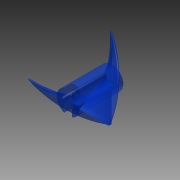
# Autodesk Inventor part: Main Prop
Saved by Autodesk Inventor 2013 (Build 170138000, 138)
## iProperties
Created: 2014-08-02
Part Number: Main Prop
Material: ABS Plastic
Document SubType Name: Modeling
Designer: Kyle
Density: 1 g/cm^3
Author: Kyle
Autodesk Inventor part; units mm, degrees
ref_plane "YZ Plane" through (0, 0, 0) normal (1, 0, 0) x (0, 1, 0)
ref_plane "XZ Plane" through (0, 0, 0) normal (0, 1, 0) x (-1, 0, 0)
sketch "Sketch1" plane through (0, 0, 0) normal (0, 0, 1) x (1, 0, 0)
  circle A0 centre (0, 0) radius 4.0005
  circle A1 centre (0, 0) radius 2.032
  dimension "d0" = 8.001
  dimension "d2" = 4.064
  constraints: 2 centre point, 2 coincident
  measures "d0" diameter of A0
  measures "d2" diameter of A1
extrude "Extrusion1" add sketch "Sketch1" along normal blind 15.24
sketch "Sketch2" plane through (0, 0, 15.24) normal (0, 0, 1) x (1, 0, 0)
  circle A0 centre (0, 0) radius 2.032 projected
  line L0 (-1.397, 5.1605) -> (1.397, 5.1605)
  line L1 (1.397, 5.1605) -> (1.397, -5.4473)
  line L2 (1.397, -5.4473) -> (-1.397, -5.4473)
  line L3 (-1.397, -5.4473) -> (-1.397, 5.1605)
  point P0 (2.032, 5.1605)
  dimension "d5" = 1.397
  dimension "d6" = 1.397
  constraints: 8 end point, 2 parallel, 1 horizontal, 1 perpendicular
  measures "d5" horizontal distance of L0.start A0.centre
  measures "d6" horizontal distance of L1.end A0.centre
extrude "Extrusion2" cut sketch "Sketch2" against normal blind 2.54 contours L1 A0 L3 | A0 L3 L0 L1 | L1 L2 L3 A0
ref_plane "Work Plane1" through (0, 0, 0) normal (0, -1, 0) x (0, 0, -1)
sketch "Sketch3" plane through (0, 0, 0) normal (0, -1, 0) x (0, 0, -1)
  line L0 (-15.24, 4.0005) -> (-15.24, 1.397) projected
  line L1 (-15.24, 4.0005) -> (-14.605, 4.0005)
  line L2 (-14.605, 4.0005) -> (-14.605, 13.9065)
  line L3 (-14.859, 14.1605) -> (-14.986, 14.1605)
  line L4 (-15.24, 13.9065) -> (-15.24, 4.0005)
  arc A0 (-14.986, 14.1605) -> (-15.24, 13.9065) centre (-14.986, 13.9065) ccw
  arc A1 (-14.605, 13.9065) -> (-14.859, 14.1605) centre (-14.859, 13.9065) ccw
  line L5 (-15.24, -4.0005) -> (-14.6794, -4.0005)
  line L6 (-14.6794, -4.0005) -> (-14.6794, -13.9065)
  line L7 (-14.9334, -14.1605) -> (-14.986, -14.1605)
  line L8 (-15.24, -13.9065) -> (-15.24, -4.0005)
  arc A2 (-15.24, -13.9065) -> (-14.986, -14.1605) centre (-14.986, -13.9065) ccw
  arc A3 (-14.9334, -14.1605) -> (-14.6794, -13.9065) centre (-14.9334, -13.9065) ccw
  point P0 (0, 0)
  point P1 (1.7022, 0)
  dimension "d10" = 4.0005
  dimension "d12" = 0.635
  dimension "d13" = 10.16
  dimension "d14" = 0.254
  dimension "d15" = 8.001
  dimension "d16" = 8.001
  dimension "d17" = 10.16
  dimension "d18" = 0.254
  constraints: 16 end point, 8 point on circle, 8 tangent, 4 centre point, 4 parallel, 2 equal radius, 2 horizontal, 2 perpendicular, 1 coincident, 1 other
  measures "d10" vertical distance of point (-14.605, 4.001) point (1.702, 0)
  measures "d12" distance from line of L0 point (-14.605, 4.001)
  measures "d13" distance between parallel lines of L3 L1
  measures "d14" radius of A0
  measures "d15" distance of L1.start L5.start
  measures "d16" vertical distance of L1.start point (-14.679, -4.001)
  measures "d17" distance between parallel lines of L5 L7
  measures "d18" radius of A2
ref_plane "Work Plane2" through (0, 0, 0) normal (-1, 0, 0) x (0, 0, -1)
sketch "Sketch4" plane through (0, 0, 0) normal (-1, 0, 0) x (0, 0, -1)
  line L0 (0, -4.0005) -> (0, 4.0005) projected
  line L1 (-1.9812, -4.0005) -> (-0.0316, -19.5002)
  line L2 (-2.54, -4.0005) -> (-0.5277, -19.5635)
  line L3 (-1.9812, -4.0005) -> (-2.54, -4.0005)
  line L4 (-0.2432, -19.7828) -> (-0.251, -19.7838)
  arc A0 (-0.5277, -19.5635) -> (-0.2432, -19.7828) centre (-0.2757, -19.5309) ccw
  arc A1 (-0.251, -19.7838) -> (-0.0316, -19.5002) centre (-0.2836, -19.5319) ccw
  line L5 (-1.9812, 4.0005) -> (-0.0317, 19.4994)
  line L6 (-2.54, 4.0005) -> (-0.5818, 19.5686)
  line L7 (-0.2981, 19.7889) -> (-0.252, 19.7831)
  arc A2 (-0.0317, 19.4994) -> (-0.252, 19.7831) centre (-0.2837, 19.5311) ccw
  arc A3 (-0.2981, 19.7889) -> (-0.5818, 19.5686) centre (-0.3298, 19.5369) ccw
  line L8 (-2.54, 4.0005) -> (-1.9812, 4.0005)
  point P0 (0, 0)
  point P1 (0.7046, 0)
  point P2 (0, -19.7514)
  point P3 (0, 19.7514)
  dimension "d25" = 15.875
  dimension "d26" = 0
  dimension "d27" = 1.9812
  dimension "d28" = 0.254
  dimension "d29" = 15.875
  dimension "d30" = 0
  dimension "d31" = 1.9812
  dimension "d32" = 0.254
  constraints: 16 end point, 8 point on circle, 8 tangent, 4 centre point, 4 point on line, 3 perpendicular, 2 equal radius, 1 parallel, 1 other
  measures "d25" distance of L1.start point (0, -19.751)
  measures "d26" horizontal distance of L0.start point (0, -19.751)
  measures "d27" distance of L1.start L0.start
  measures "d28" radius of A0
  measures "d29" distance of L5.start point (0, 19.751)
  measures "d30" distance from line of point (0, 19.751) L0
  measures "d31" distance from line of L5.start L0
  measures "d32" radius of A2
coil "Coil1" sketch "Sketch3" operation add axis through (0, 0, 0) along (0, 0, -1) pitch 58.42 turns 0.25 hand left contours L4 A0 L3 A1 L2 L1
coil "Coil2" sketch "Sketch3" operation add axis through (0, 0, 0) along (0, 0, -1) pitch 58.42 turns 0.25 hand left contours L5 L6 A3 L7 A2 L8
body "Solid1"
